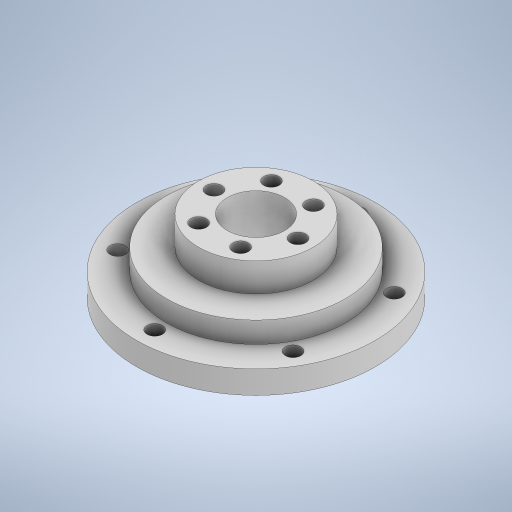
# Autodesk Inventor part: OnPatronFlanech
Saved by Autodesk Inventor 2024 (Build 280153000, 153)
## iProperties
Created: 2023-08-26
Part Number: OnPatronFlanech
Material: Generic
Document SubType Name: Modeling
Designer: KirikDK
Density: 1 g/cm^3
Appearance: Default
Author: KirikDK
Autodesk Inventor part; units mm, degrees
ref_plane "YZ Plane" through (0, 0, 0) normal (1, 0, 0) x (0, 1, 0)
ref_plane "XZ Plane" through (0, 0, 0) normal (0, 1, 0) x (-1, 0, 0)
ref_plane "XY Plane" through (0, 0, 0) normal (0, 0, 1) x (1, 0, 0)
sketch "Sketch1" plane through (0, 0, 0) normal (0, 1, 0) x (-1, 0, 0)
  circle A0 centre (0, 0) radius 62.5
  circle A1 centre (0, 0) radius 53
  circle A2 centre (0, -53) radius 4.05
  circle A3 centre (0, 0) radius 44
  circle A4 centre (45.8993, -26.5) radius 4.05
  circle A5 centre (45.8993, 26.5) radius 4.05
  circle A6 centre (0, 53) radius 4.05
  circle A7 centre (-45.8993, 26.5) radius 4.05
  circle A8 centre (-45.8993, -26.5) radius 4.05
  dimension "d1" = 106
  dimension "d0" = 125
  dimension "d4" = 360
  dimension "d18" = 8.1
  constraints: 8 centre point, 3 coincident, 1 vertical alignment, 15 other
  measures "d0" diameter of A0
  measures "d18" diameter of A2
extrude "Extrusion1" add sketch "Sketch1" along normal blind 12 contours A0 | A1 A4 A2 A8 A7 A6 A5
sketch "Sketch2" plane through (0, 12, 0) normal (0, 1, 0) x (1, 0, 0)
  circle A0 centre (0, 0) radius 44 projected
  circle A1 centre (0, 0) radius 15
  circle A2 centre (-22, 0) radius 4.05
  circle A3 centre (-11, -19.0526) radius 4.05
  circle A4 centre (11, -19.0526) radius 4.05
  circle A5 centre (22, 0) radius 4.05
  circle A6 centre (11, 19.0526) radius 4.05
  circle A7 centre (-11, 19.0526) radius 4.05
  dimension "d8" = 30
  dimension "d11" = 22
  dimension "d12" = 8.1
  dimension "d15" = 360
  constraints: 7 centre point, 1 coincident, 13 other
  measures "d8" diameter of A1
  measures "d11" distance of point (0, 0) A2.centre
  measures "d12" diameter of A2
extrude "Extrusion2" add sketch "Sketch2" against normal blind 8
sketch "Sketch3" plane through (0, 12, 0) normal (0, 1, 0) x (1, 0, 0)
  circle A0 centre (0, 0) radius 30
  circle A1 centre (0, 0) radius 15 projected
  circle A2 centre (-22, 0) radius 4.05 projected
  circle A3 centre (-11, -19.0526) radius 4.05 projected
  circle A4 centre (11, -19.0526) radius 4.05 projected
  circle A5 centre (22, 0) radius 4.05 projected
  circle A6 centre (11, 19.0526) radius 4.05 projected
  circle A7 centre (-11, 19.0526) radius 4.05 projected
  circle A8 centre (0, 0) radius 62.5 projected
  circle A9 centre (0, 53) radius 4.05 projected
  circle A10 centre (-45.8993, 26.5) radius 4.05 projected
  circle A11 centre (-45.8993, -26.5) radius 4.05 projected
  circle A12 centre (0, -53) radius 4.05 projected
  circle A13 centre (45.8993, -26.5) radius 4.05 projected
  circle A14 centre (45.8993, 26.5) radius 4.05 projected
  dimension "d17" = 60
  constraints: 1 centre point, 1 coincident
  measures "d17" diameter of A0
extrude "Extrusion3" add sketch "Sketch3" along normal blind 24 contours A0
sketch "Sketch4" plane through (0, 12, 0) normal (0, 1, 0) x (1, 0, 0)
  circle A0 centre (0, 0) radius 46.75
  circle A1 centre (0, 0) radius 44 projected
  circle A2 centre (0, 0) radius 30 projected
  circle A3 centre (0, 0) radius 62.5 projected
  circle A4 centre (0, 53) radius 4.05 projected
  circle A5 centre (-45.8993, 26.5) radius 4.05 projected
  circle A6 centre (-45.8993, -26.5) radius 4.05 projected
  circle A7 centre (0, -53) radius 4.05 projected
  circle A8 centre (45.8993, -26.5) radius 4.05 projected
  circle A9 centre (45.8993, 26.5) radius 4.05 projected
  dimension "d24" = 93.5
  constraints: 1 centre point, 1 coincident
  measures "d24" diameter of A0
extrude "Extrusion4" add sketch "Sketch4" along normal blind 11 contours A0 | A1
sketch "Sketch5" plane through (0, 36, 0) normal (0, 1, 0) x (1, 0, 0)
  circle A0 centre (0, 0) radius 30 projected
  circle A1 centre (-11, 19.0526) radius 4.05 projected
  circle A2 centre (11, 19.0526) radius 4.05 projected
  circle A3 centre (22, 0) radius 4.05 projected
  circle A4 centre (11, -19.0526) radius 4.05 projected
  circle A5 centre (-11, -19.0526) radius 4.05 projected
  circle A6 centre (-22, 0) radius 4.05 projected
  circle A7 centre (0, 0) radius 15 projected
extrude "Extrusion5" add sketch "Sketch5" along normal blind 2
body "Solid1"
